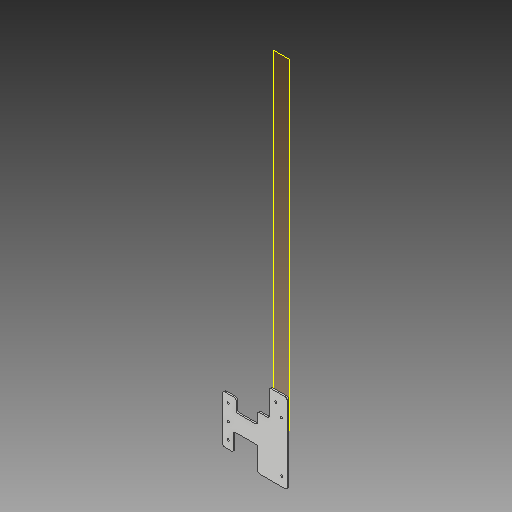
# Autodesk Inventor part: Part1
Saved by Autodesk Inventor 2018 (Build 220112000, 112)
## iProperties
Created: 2017-06-06
Part Number: Part1
Material: Generic
Document SubType Name: Modeling
Designer: m228540
Density: 1 g/cm^3
Appearance: Default
Author: m228540
Autodesk Inventor part; units mm, degrees
ref_plane "YZ Plane" through (0, 0, 0) normal (1, 0, 0) x (0, 1, 0)
ref_plane "XZ Plane" through (0, 0, 0) normal (0, 1, 0) x (-1, 0, 0)
ref_plane "XY Plane" through (0, 0, 0) normal (0, 0, 1) x (1, 0, 0)
ref_plane "Work Plane1" through (678.6266, 4, 0) normal (0, 0, 1) x (1, 0, 0)
sketch "Sketch1" plane through (678.6266, 4, 0) normal (0, 0, 1) x (1, 0, 0)
  line L0 (0.5726, -1046.8384) -> (-66.4274, -1046.8384)
  line L1 (-109.4274, -1346.8384) -> (0.5726, -1346.8384)
  line L2 (0.5726, -1346.8384) -> (0.5726, -1046.8384)
  line L3 (-109.4274, -1256.8384) -> (-201.4274, -1256.8384)
  line L4 (-201.4274, -1256.8384) -> (-201.4274, -1324.8384)
  line L5 (-201.4274, -1324.8384) -> (-241.4274, -1324.8384)
  line L6 (-241.4274, -1324.8384) -> (-241.4274, -1144.8384)
  line L7 (-191.4274, -1190.8384) -> (-111.4274, -1190.8384)
  line L8 (-111.4274, -1146.8384) -> (-111.4274, -1190.8384)
  line L9 (-109.4274, -1256.8384) -> (-109.4274, -1346.8384)
  line L10 (-241.4274, -1144.8384) -> (-191.4274, -1144.8384)
  line L11 (-191.4274, -1144.8384) -> (-191.4274, -1190.8384)
  line L12 (-111.4274, -1146.8384) -> (-66.4274, -1146.8384)
  line L13 (-66.4274, -1146.8384) -> (-66.4274, -1046.8384)
  point P0 (-678.6266, -4)
  dimension "d0" = 110
  dimension "d4" = 92
  dimension "d5" = 68
  dimension "d6" = 40
  dimension "d7" = 180
  dimension "d8" = 50
  dimension "d9" = 46
  dimension "d10" = 300
  dimension "d12" = 80
  dimension "d13" = 44
  dimension "d14" = 45
  dimension "d15" = 100
  constraints: 28 end point, 11 perpendicular, 3 horizontal, 3 parallel
  measures "d0" distance of L1.start L1.end
  measures "d4" distance of L3.start L3.end
  measures "d5" distance of L3.end L4.end
  measures "d6" distance of L4.end L5.end
  measures "d7" distance of L5.end L6.end
  measures "d8" distance of L6.end L10.end
  measures "d9" distance of L10.end L7.start
  measures "d10" distance of L1.end L0.start
  measures "d12" distance of L7.start L7.end
  measures "d13" distance of L8.start L7.end
  measures "d14" distance of L8.start L12.end
  measures "d15" distance of L12.end L0.end
extrude "Extrusion1" add sketch "Sketch1" along normal blind 6
fillet "Fillet1" radius 7 14 edges at (487.1992, -1186.8384, 3) (567.1992, -1186.8384, 3) (612.1992, -1042.8384, 3) (679.1992, -1042.8384, 3) (487.1992, -1140.8384, 3) (437.1992, -1140.8384, 3) (437.1992, -1320.8384, 3) (477.1992, -1320.8384, 3) (477.1992, -1252.8384, 3) (569.1992, -1252.8384, 3) (569.1992, -1342.8384, 3) (679.1992, -1342.8384, 3) (567.1992, -1142.8384, 3) (612.1992, -1142.8384, 3)
sketch "Sketch2" plane through (678.6266, 4, 6) normal (0, 0, 1) x (1, 0, 0)
  circle A0 centre (-221.4274, -1294.8384) radius 4
  circle A1 centre (-221.4274, -1234.8384) radius 4
  circle A2 centre (-221.4274, -1174.8384) radius 4
  line L0 (-234.4274, -1324.8384) -> (-208.4274, -1324.8384) projected
  line L1 (-221.4274, -1324.8384) -> (-221.4274, -1294.8384) construction
  line L2 (-221.4274, -1294.8384) -> (-221.4274, -1234.8384) construction
  line L3 (-221.4274, -1234.8384) -> (-221.4274, -1174.8384) construction
  line L4 (-241.4274, -1151.8384) -> (-241.4274, -1317.8384) projected
  line L5 (-241.4274, -1234.8384) -> (-221.4274, -1234.8384) construction
  circle A3 centre (-19.4274, -1311.8384) radius 4
  circle A4 centre (-21.4274, -1121.8384) radius 4
  circle A5 centre (-41.4274, -1081.8384) radius 4
  line L6 (-102.4274, -1346.8384) -> (-6.4274, -1346.8384) projected
  line L7 (0.5726, -1339.8384) -> (0.5726, -1053.8384) projected
  line L8 (-6.4274, -1046.8384) -> (-59.4274, -1046.8384) projected
  line L9 (-66.4274, -1053.8384) -> (-66.4274, -1139.8384) projected
  point P0 (-678.6266, -4)
  dimension "d17" = 8
  dimension "d18" = 60
  dimension "d19" = 60
  dimension "d20" = 8
  dimension "d21" = 35
  dimension "d22" = 20
  dimension "d23" = 35
  dimension "d24" = 25
  dimension "d25" = 40
  dimension "d26" = 20
  dimension "d27" = 30
  constraints: 8 end point, 6 centre point, 4 equal radius, 2 collinear, 2 midpoint, 1 perpendicular
  measures "d17" diameter of A0
  measures "d18" distance of L2.end L3.end
  measures "d19" distance of L1.end L2.end
  measures "d20" diameter of A3
  measures "d21" distance from line of L6 A3.centre
  measures "d22" distance from line of L7 A3.centre
  measures "d23" distance from line of L8 A5.centre
  measures "d24" distance from line of L9 A5.centre
  measures "d25" vertical distance of A5.centre A4.centre
  measures "d26" horizontal distance of A5.centre A4.centre
  measures "d27" distance of L1.start L1.end
extrude "Extrusion2" cut sketch "Sketch2" against normal through all
body "Solid1"
